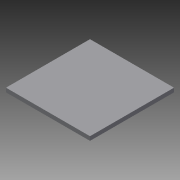
# Autodesk Inventor part: plane
Saved by Autodesk Inventor 2015 (Build 190159000, 159)
## iProperties
Created: 2016-11-24
Part Number: plane
Material: Generic
Document SubType Name: Modeling
Designer: Eduard
Density: 1 g/cm^3
Appearance: Default
Author: Eduard
Autodesk Inventor part; units mm, degrees
ref_plane "YZ Plane" through (0, 0, 0) normal (1, 0, 0) x (0, 1, 0)
ref_plane "XZ Plane" through (0, 0, 0) normal (0, 1, 0) x (-1, 0, 0)
ref_plane "XY Plane" through (0, 0, 0) normal (0, 0, 1) x (1, 0, 0)
sketch "Sketch1" plane through (0, 0, 0) normal (0, 0, 1) x (1, 0, 0)
  line L0 (-9.2658, 8.8818) -> (11.723, 8.8818)
  line L1 (11.723, 8.8818) -> (11.723, -12.1069)
  line L2 (11.723, -12.1069) -> (-9.2658, -12.1069)
  line L3 (-9.2658, -12.1069) -> (-9.2658, 8.8818)
  point P0 (0, 0)
  constraints: 8 end point, 2 parallel, 1 horizontal, 1 perpendicular
extrude "Extrusion1" add sketch "Sketch1" along normal blind 1
body "Solid1"
